Faucet Straightener (Autodesk Fusion 360 design; units mm, degrees)
Autodesk Fusion 360 part; units mm, degrees
note: some values were not read from the file. Set by a fixed rule: which sketch regions a step uses.
sketch "Sketch1" plane through (0, 0, 0) normal (0, 0, 1) x (1, 0, 0)
  circle A0 centre (0, 0) radius 10
  dimension "d1" = 20
  constraint coincident A0.centre origin
  measures "d1" diameter of A0
sketch "Sketch2" plane through (0, 0, 0) normal (0, 0, 1) x (1, 0, 0)
  circle A0 centre (0, 0) radius 17.5
  circle A1 centre (0, 0) radius 14
  line L0 (-0.75, 19.1081) -> (0.75, 19.1081)
  line L1 (0.75, 19.1081) -> (0.75, -21)
  line L2 (0.75, -21) -> (-0.75, -21)
  line L3 (-0.75, -21) -> (-0.75, 19.1081)
  line L4 (0, 23) -> (0, -27)
  line L5 (-30, 0) -> (27, 0)
  line L6 (-16.3017, -8.5458) -> (18.0876, 11.3089)
  line L7 (18.0876, 11.3089) -> (18.8376, 10.0099)
  line L8 (18.8376, 10.0099) -> (-15.5517, -9.8448)
  line L9 (-15.5517, -9.8448) -> (-16.3017, -8.5458)
  line L10 (-16.8985, 10.6224) -> (17.4908, -9.2323)
  line L11 (17.4908, -9.2323) -> (16.7408, -10.5313)
  line L12 (16.7408, -10.5313) -> (-17.6485, 9.3234)
  line L13 (-17.6485, 9.3234) -> (-16.8985, 10.6224)
  line L14 (8.0661, -18.0086) -> (4.1738, -11.2669)
  line L15 (4.1738, -11.2669) -> (8.0709, -9.0169)
  line L16 (8.0709, -9.0169) -> (11.9633, -15.7586)
  line L17 (11.9633, -15.7586) -> (8.0661, -18.0086)
  dimension "d2" = 35
  dimension "d3" = 28
  dimension "d4" = 1.5
  dimension "d5" = 0.75
  dimension "d7" = 1.5
  dimension "d8" = 120
  dimension "d9" = 0.75
  dimension "d10" = 1.5
  dimension "d11" = 60
  dimension "d16" = 4.5
  dimension "d17" = 30
  dimension "d19" = 0.75
  constraint coincident A0.centre A1.centre
  constraint horizontal L0
  constraint vertical L1
  constraint horizontal L2
  constraint vertical L3
  constraint perpendicular L4 L5
  constraint perpendicular L6 L7
  constraint parallel L6 L8
  constraint parallel L7 L9
  constraint perpendicular L10 L11
  constraint parallel L10 L12
  constraint parallel L11 L13
  constraint perpendicular L14 L15
  constraint parallel L14 L16
  constraint parallel L15 L17
  measures "d2" diameter of A0
  measures "d3" diameter of A1
  measures "d4" distance of L0.start L0.end
  measures "d5" distance of L1 A0.centre
  measures "d7" distance of L6.start L8.end
  measures "d8" angle of L4 L6
  measures "d9" distance of A0.centre L6
  measures "d10" distance of L10.start L12.end
  measures "d11" angle of L4 L10
  measures "d16" distance of L14.start L16.end
  measures "d17" angle of L4 L14
  measures "d19" distance of A0.centre L12
extrude "Extrude1" add sketch "Sketch2" along normal blind 200 contours A0 A1 L5 L8 | A0 A1 L5 L10 | A0 A1 L6 L8 | A0 A1 L10 L12 | A0 A1 L1 L6 | A0 A1 L12 L16 | A0 A1 L1 L4 | A0 A1 L3 L4 | A0 A1 L1 L14 | A0 A1 L3 L10 | A0 A1 L1 L4 | A0 A1 L3 L4 | A0 A1 L10 L12 | A0 A1 L3 L8 | A0 A1 L6 L8 | A0 A1 L5 L12 | A0 A1 L5 L6
extrude "Extrude2" cut sketch "Sketch2" along normal blind 6 contours A0 A1 L6 L8 | A0 A1 L10 L12 | A0 A1 L1 L4 | A0 A1 L3 L4 | A0 A1 L1 L4 | A0 A1 L3 L4 | A0 A1 L10 L12 | A0 A1 L6 L8
sketch "Sketch3" plane through (0, 0, 200) normal (0, 0, 1) x (-1, 0, 0)
  arc A0 (-10.8104, 13.7617) -> (-6.9432, 16.0637) centre (0, 0) ccw
  line L0 (-6.9432, 16.0637) -> (-5.1785, 13.007)
  arc A1 (-9.038, 10.6918) -> (-5.1785, 13.007) centre (0, 0) ccw
  line L1 (-9.038, 10.6918) -> (-10.8104, 13.7617)
  line L2 (-17.6603, 9.8038) -> (-17.3205, -10.3923)
  line L3 (-17.3205, -10.3923) -> (0.3397, -20.1962)
  line L4 (0.3397, -20.1962) -> (17.6603, -9.8038)
  line L5 (17.6603, -9.8038) -> (17.3205, 10.3923)
  line L6 (17.3205, 10.3923) -> (-0.3397, 20.1962)
  line L7 (-0.3397, 20.1962) -> (-17.6603, 9.8038)
  line L8 (-6.6088, 16.4347) -> (-6.9432, 16.0637)
  line L9 (-10.8104, 13.7617) -> (-11.4119, 13.5528)
  constraint coincident A0.centre A1.centre
  constraint coincident L7 L8.start
  constraint coincident A0.end L0.start
  constraint coincident A0.start L1.end
  constraint coincident L7 L9.end
extrude "Extrude3" add sketch "Sketch3" against normal blind 40 contours A0 L2 L7 L9 | A0 L2 L3 | A0 L6 L7 L8 | A0 L3 L4 | A0 L5 L6 | A0 L4 L5
